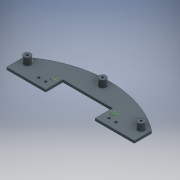
# Autodesk Inventor part: Base
Saved by Autodesk Inventor 2017 SP1 (Build 210196100, 196)
## iProperties
Created: 2017-05-08
Part Number: Base
Material: ABS Plastic
Document SubType Name: Modeling
Designer: zallen
Density: 1.06 g/cm^3
Appearance: CR Dark Blue
Mass: 72.8492 g
Surface Area: 267.673 cm^2
Volume: 68.7257 cm^3
Author: zallen
Autodesk Inventor part; units mm, degrees
ref_plane "YZ Plane" through (0, 0, 0) normal (1, 0, 0) x (0, 1, 0)
ref_plane "XZ Plane" through (0, 0, 0) normal (0, 1, 0) x (-1, 0, 0)
ref_plane "XY Plane" through (0, 0, 0) normal (0, 0, 1) x (1, 0, 0)
sketch "Sketch1" plane through (0, 0, 0) normal (0, 0, 1) x (1, 0, 0)
  line L0 (0, 0) -> (0, -85) construction
  line L1 (-139.0912, -85) -> (-139.0912, -47.1845)
  arc A0 (0, 0) -> (-139.0912, -47.1845) centre (0.0113, -228.6333) ccw
  circle A1 centre (0, -15) radius 7.5
  circle A2 centre (-124.0912, -55) radius 7.5
  line L2 (-124.4333, -85) -> (-76.2679, -85) construction
  line L3 (139.0912, -85) -> (139.0912, -47.1845)
  arc A3 (139.0912, -47.1845) -> (0, 0) centre (-0.0113, -228.6333) ccw
  circle A4 centre (124.0912, -55) radius 7.5
  line L4 (124.4333, -85) -> (124.4333, -36.8346) construction
  line L5 (-139.0912, -85) -> (-54.0912, -85)
  line L6 (139.0912, -85) -> (54.0912, -85)
  line L7 (-54.0912, -85) -> (-54.0912, -47.5)
  line L8 (-54.0912, -47.5) -> (54.0912, -47.5)
  line L9 (54.0912, -47.5) -> (54.0912, -85)
  dimension "d45" = 15
  dimension "d46" = 15
  dimension "d47" = 15
  dimension "d48" = 15
  dimension "d51" = 139.0912
  dimension "d54" = 228.6333
  dimension "d55" = 85
  dimension "d58" = 139.1025
  dimension "d110" = 85
  dimension "d111" = 85
  dimension "d112" = 181.1333
  dimension "d114" = 85
  dimension "d130" = 108.1825
  constraints: 20 end point, 5 centre point, 5 point on circle, 5 symmetric about line, 2 horizontal, 2 perpendicular, 2 vertical, 1 point on line, 2 other
  measures "d45" diameter of A1
  measures "d46" distance of A1.centre L0.start
  measures "d47" diameter of A2
  measures "d48" distance from line of L1 A2.centre
  measures "d51" distance between parallel lines of L0 L1
  measures "d54" radius of A3
  measures "d55" distance of L0.start L0.end
  measures "d58" distance from line of A0.centre L1
  measures "d110" distance of L1.start L5.end
  measures "d111" distance of L3.start L6.end
  measures "d112" distance from line of A3.centre L8
  measures "d114" distance from line of L0.start L5
  measures "d130" distance between parallel lines of L9 L7
extrude "Extrusion4" add sketch "Sketch1" along normal blind 5
sketch "Sketch4" plane through (0, 0, 5) normal (0, 0, 1) x (1, 0, 0)
  circle A0 centre (-124.0912, -55) radius 7.5 projected
  circle A1 centre (-124.0912, -55) radius 7.5
  circle A2 centre (0, -15) radius 7.5 projected
  circle A3 centre (0, -15) radius 7.5
  circle A4 centre (124.0912, -55) radius 7.5 projected
  circle A5 centre (124.0912, -55) radius 7.5
  point P0 (0, 0)
  constraints: 3 centre point, 3 coincident
extrude "Extrusion5" add sketch "Sketch4" along normal mid plane 10
sketch "Sketch5" plane through (0, 0, 5) normal (0, 0, 1) x (1, 0, 0)
  circle A0 centre (-124.0912, -55) radius 7.5 projected
  circle A1 centre (-124.0912, -55) radius 7.5
  circle A2 centre (-124.0912, -55) radius 7.5
  circle A3 centre (0, -15) radius 7.5 projected
  circle A4 centre (0, -15) radius 7.5
  circle A5 centre (124.0912, -55) radius 7.5 projected
  circle A6 centre (124.0912, -55) radius 7.5
  point P0 (0, 0)
  constraints: 4 centre point, 4 coincident
extrude "Extrusion6" add sketch "Sketch5" along normal blind 15
sketch "Sketch7" plane through (0, 0, 5) normal (0, 0, 1) x (1, 0, 0)
  circle A0 centre (-69.0912, -60) radius 1
  circle A1 centre (-62.6912, -60) radius 1
  line L0 (-139.0912, -47.1845) -> (-139.0912, -85) projected
  line L1 (0, -85) -> (0, 2.05) construction
  line L2 (-139.0912, -85) -> (-54.0912, -85) construction
  line L3 (-139.0912, -85) -> (0, -85) construction
  circle A2 centre (69.0912, -60) radius 1
  circle A3 centre (62.6912, -60) radius 1
  point P0 (0, 0)
  dimension "d72" = 2
  dimension "d73" = 2
  dimension "d74" = 6.4
  dimension "d76" = 70
  dimension "d115" = 25
  constraints: 4 centre point, 4 end point, 2 symmetric about line, 1 collinear, 1 horizontal alignment, 1 vertical, 2 other
  measures "d72" diameter of A0
  measures "d73" diameter of A1
  measures "d74" distance of A1.centre A0.centre
  measures "d76" distance from line of L0 A0.centre
  measures "d115" distance from line of L2 A0.centre
extrude "Extrusion11" cut sketch "Sketch7" against normal through all
thread "Thread7" size "M2x0.4" class "6H" standard "ISO Metric profile" full length
thread "Thread8" size "M2x0.4" class "6H" standard "ISO Metric profile" full length
thread "Thread9" size "M2x0.4" class "6H" standard "ISO Metric profile" full length
thread "Thread10" size "M2x0.4" class "6H" standard "ISO Metric profile" full length
sketch "Sketch8" plane through (0, 0, 5) normal (0, 0, 1) x (1, 0, 0)
  point P0 (-62.6912, -55)
sketch "Sketch9" plane through (0, 0, 5) normal (0, 0, 1) x (1, 0, 0)
  point P0 (69.0912, -55)
sketch "Sketch10" plane through (0, 0, 5) normal (0, 0, 1) x (1, 0, 0)
  point P0 (62.6912, -55)
sketch "Sketch11" plane through (0, 0, 5) normal (0, 0, 1) x (1, 0, 0)
  point P0 (62.6912, -55)
hole "Hole6" at (62.6912, -55, 5) direction (0, 0, -1) diameter 1.567 depth 6.2 tip angle 120 thread size "M2x0.4" class "6H" standard "ISO Metric profile"
sketch "Sketch12" plane through (0, 0, 5) normal (0, 0, 1) x (1, 0, 0)
  point P0 (69.0912, -55)
hole "Hole8" at (69.0912, -55, 5) direction (0, 0, -1) diameter 1.567 depth 6.2 tip angle 120 thread size "M2x0.4" class "6H" standard "ISO Metric profile"
sketch "Sketch13" plane through (0, 0, 5) normal (0, 0, 1) x (1, 0, 0)
  circle A0 centre (-84.0912, -70) radius 2.5
  circle A1 centre (-69.0912, -70) radius 2.5
  line L0 (-139.0912, -85) -> (-54.0912, -85) projected
  line L1 (-54.0912, -85) -> (-54.0912, -47.5) projected
  arc A2 (0, 0) -> (-139.0912, -47.1845) centre (0.0113, -228.6333) ccw construction
  line L2 (0, 0) -> (0, -107.8071) construction
  circle A3 centre (84.0912, -70) radius 2.5
  circle A4 centre (69.0912, -70) radius 2.5
  dimension "d145" = 5
  dimension "d146" = 5
  dimension "d147" = 15
  dimension "d148" = 15
  dimension "d149" = 15
  constraints: 4 centre point, 2 end point, 2 symmetric about line, 1 horizontal alignment, 1 vertical, 2 other
  measures "d145" diameter of A0
  measures "d146" diameter of A1
  measures "d147" distance from line of L0 A1.centre
  measures "d148" distance from line of L1 A1.centre
  measures "d149" distance of A1.centre A0.centre
extrude "Extrusion12" cut sketch "Sketch13" against normal through all
sketch "Sketch14" plane through (0, -15, 20) normal (0, 0, 1) x (1, 0, 0)
  circle A0 centre (0, 0) radius 2.5
  circle A1 centre (-124.0912, -40) radius 7.5 construction
  circle A2 centre (0, 0) radius 7.5 construction
  circle A3 centre (124.0912, -40) radius 7.5 construction
  circle A4 centre (-124, -40) radius 2.5
  circle A5 centre (124, -40) radius 2.5
  point P0 (0, 15)
  dimension "d152" = 5
  dimension "d155" = 5
  dimension "d156" = 5
  dimension "d157" = 40
  dimension "d158" = 124
  dimension "d159" = 124
  dimension "d160" = 40
  constraints: 3 centre point, 1 coincident
  measures "d152" diameter of A0
  measures "d155" diameter of A4
  measures "d156" diameter of A5
  measures "d157" vertical distance of A0.centre A5.centre
  measures "d158" horizontal distance of A5.centre A0.centre
  measures "d159" horizontal distance of A0.centre A4.centre
  measures "d160" vertical distance of A0.centre A4.centre
extrude "Extrusion13" cut sketch "Sketch14" against normal blind 10
thread "Thread11" size "M5x0.8" class "6H" standard "ISO Metric profile" full length
thread "Thread12" size "M5x0.8" class "6H" standard "ISO Metric profile" full length
thread "Thread13" size "M5x0.8" class "6H" standard "ISO Metric profile" full length
body "Solid2"
